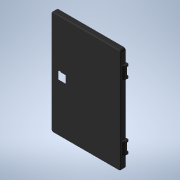
# Autodesk Inventor part: 1301.000_2_(1)
Saved by Autodesk Inventor 2021 (Build 250183000, 183)
## iProperties
Created: 2025-05-02
Part Number: 1301.000_2_(1)
Material: Generic
Catalog Web Link: www.cadenas.de
Description: Deckel KX EB Edelstahl-Deckel KX EB Edelstahl
Vendor: RITTAL
Document SubType Name: Modeling
Designer: psAdmin
Manufacturer: RITTAL
Mass: 142.258 g
Surface Area: 1510.1 cm^2
Volume: 142.258 cm^3
Density: 1 g/cm^3
Appearance: PSOLRGB-175-175-175
Category: PARTsolutions
Company: RITTAL
Title: 1301.000_2
Author: Cadenas PARTsolutions
Comments: Deckel KX EB Edelstahl
PSOL_IDENT_0: {$CADENAS_DATA/23d-libs/rittal/schaltschranksys/edelstahl/kleingehause/parts_eb_edel_2_0/deckel_kx_e
PSOL_IDENT_1: b_edel_new.prj},193 {VTYP=3D},{NB=1301.000_2_(1)},{LINA=1301.000_2},{NN=Deckel KX EB Edelstahl},{DAT
PSOL_IDENT_2: E=28.04.2025 21:10:47},{GEOMDATE=11.04.2025 11:21:28},{VERSION=},{LINEID=690},{WBVAR=DETAIL},{WBNUME
PSOL_IDENT_3: RIC=DETAIL}  {NB=1301.000_2_(1)},{LINA=1301.000_2},{KT=DUMMY},{BEST=1301.000},{DETAIL=1},{B=200},{H=
PSOL_IDENT_4: 300},{W=198.000},{H1=298.000},{A1=167.450},{GEW=3,889},{S1=1.250},{CNSETIM80=EC000261},{CNSETIM90=EC
PSOL_IDENT_5: 000261},{CNSECLASS60=27-18-01-01},{CNSECLASS80=27-18-01-01},{UNSPSC=31-26-15-02}
NB: 1301.000_2_(1)
NN: Deckel KX EB Edelstahl
NT: Deckel KX EB Edelstahl
NBSYN: $BEST._2_($DETAIL.)
LINA: 1301.000_2
CATALOG: Rittal
BEST: 1301.000
DETAIL: hoch
B: 200
H: 300
W: 198
H1: 298
A1: 167.45
GEW: 3,889
S1: 1.25
CNSETIM80: EC000261
CNSETIM90: EC000261
CNSECLASS60: 27-18-01-01
CNSECLASS80: 27-18-01-01
UNSPSC: 31-26-15-02
SUPPLIER: RITTAL
ARTICLENO: 1301.000_2_(1)
BOMINFO: 1301.000_2
CREATOR: CADENAS GmbH
Autodesk Inventor part; units mm, degrees
ref_plane "YZ Plane" through (0, 0, 0) normal (1, 0, 0) x (0, 1, 0)
ref_plane "XZ Plane" through (0, 0, 0) normal (0, 1, 0) x (-1, 0, 0)
ref_plane "XY Plane" through (0, 0, 0) normal (0, 0, 1) x (1, 0, 0)
sketch "Skizze_2" plane through (0, 0, 0) normal (1, 0, 0) x (0, 0, -1)
  line L0 (0, -149) -> (15, -149)
  line L1 (15, -149) -> (15, -147.75)
  line L2 (15, -147.75) -> (1.25, -147.75)
  line L3 (1.25, -147.75) -> (1.25, 147.75)
  line L4 (1.25, 147.75) -> (15, 147.75)
  line L5 (15, 147.75) -> (15, 149)
  line L6 (15, 149) -> (0, 149)
  line L7 (0, 149) -> (0, -149)
  constraints: 16 end point
extrude "Extrusion1" add sketch "Skizze_2" along normal mid plane 186
sketch "Skizze_4" plane through (0, 0, 0) normal (0, 1, 0) x (1, 0, 0)
  line L0 (-99, 15) -> (-99, 0)
  line L1 (-99, 0) -> (99, 0)
  line L2 (99, 0) -> (99, 15)
  line L3 (99, 15) -> (97.75, 15)
  line L4 (97.75, 15) -> (97.75, 1.25)
  line L5 (97.75, 1.25) -> (-97.75, 1.25)
  line L6 (-97.75, 1.25) -> (-97.75, 15)
  line L7 (-97.75, 15) -> (-99, 15)
  constraints: 16 end point
extrude "Extrusion2" add sketch "Skizze_4" along normal mid plane 286
sketch "Skizze_5" plane through (0, 143, 0) normal (0, 1, 0) x (1, 0, 0)
  line L0 (93, 0) -> (93, 1.25)
  line L1 (93, 1.25) -> (97.75, 1.25)
  line L2 (97.75, 1.25) -> (97.75, 15)
  line L3 (97.75, 15) -> (99, 15)
  line L4 (99, 15) -> (99, 2.5)
  arc A0 (96.5, 0) -> (99, 2.5) centre (96.5, 2.5) ccw
  line L5 (96.5, 0) -> (93, 0)
  line L6 (93, 0) -> (93, 1.25)
  constraints: 14 end point, 2 point on circle, 1 centre point
revolve "Revolution1" add sketch "Skizze_5" angle 90 about axis through (93, 143, 0) along (0, 0, 1)
sketch "Skizze_6" plane through (0, 143, 0) normal (0, 1, 0) x (1, 0, 0)
  line L0 (-93, 1.25) -> (-93, 0)
  line L1 (-93, 0) -> (-96.5, 0)
  arc A0 (-99, 2.5) -> (-96.5, 0) centre (-96.5, 2.5) ccw
  line L2 (-99, 2.5) -> (-99, 15)
  line L3 (-99, 15) -> (-97.75, 15)
  line L4 (-97.75, 15) -> (-97.75, 1.25)
  line L5 (-97.75, 1.25) -> (-93, 1.25)
  line L6 (-93, 1.25) -> (-93, 0)
  constraints: 14 end point, 2 point on circle, 1 centre point
revolve "Revolution2" add sketch "Skizze_6" angle 90 about axis through (-93, 143, -1.25) along (0, 0, -1)
sketch "Skizze_7" plane through (0, -143, 0) normal (0, 1, 0) x (1, 0, 0)
  line L0 (93, 0) -> (93, 1.25)
  line L1 (93, 1.25) -> (97.75, 1.25)
  line L2 (97.75, 1.25) -> (97.75, 15)
  line L3 (97.75, 15) -> (99, 15)
  line L4 (99, 15) -> (99, 2.5)
  arc A0 (96.5, 0) -> (99, 2.5) centre (96.5, 2.5) ccw
  line L5 (96.5, 0) -> (93, 0)
  line L6 (93, 0) -> (93, 1.25)
  constraints: 14 end point, 2 point on circle, 1 centre point
revolve "Revolution3" add sketch "Skizze_7" angle 90 about axis through (93, -143, 0) along (0, 0, -1)
sketch "Skizze_8" plane through (0, -143, 0) normal (0, 1, 0) x (1, 0, 0)
  line L0 (-93, 1.25) -> (-93, 0)
  line L1 (-93, 0) -> (-96.5, 0)
  arc A0 (-99, 2.5) -> (-96.5, 0) centre (-96.5, 2.5) ccw
  line L2 (-99, 2.5) -> (-99, 15)
  line L3 (-99, 15) -> (-97.75, 15)
  line L4 (-97.75, 15) -> (-97.75, 1.25)
  line L5 (-97.75, 1.25) -> (-93, 1.25)
  line L6 (-93, 1.25) -> (-93, 0)
  constraints: 14 end point, 2 point on circle, 1 centre point
revolve "Revolution4" add sketch "Skizze_8" angle 90 about axis through (-93, -143, -1.25) along (0, 0, 1)
sketch "Skizze_29" plane through (0, 0, 0) normal (1, 0, 0) x (0, 0, -1)
  line L0 (0, 147.75) -> (0, -147.75)
  line L1 (0, -147.75) -> (1.25, -147.75)
  arc A0 (1.25, -147.75) -> (1.25, -136.75) centre (1.7292, -142.25) ccw
  line L2 (1.25, -136.75) -> (1.25, 136.75)
  arc A1 (1.25, 136.75) -> (1.25, 147.75) centre (1.7292, 142.25) ccw
  line L3 (1.25, 147.75) -> (0, 147.75)
  constraints: 8 end point, 4 point on circle, 2 centre point
extrude "Extrusion3" add sketch "Skizze_29" along normal mid plane 176.5
sketch "Skizze_30" plane through (88.25, 0, 0) normal (1, 0, 0) x (0, 0, -1)
  line L0 (5.5344, 138.25) -> (1.25, 138.25)
  line L1 (1.25, 138.25) -> (1.25, 147.7708)
  line L2 (1.25, 147.7708) -> (1.7292, 147.7708)
  arc A0 (5.5344, 138.25) -> (1.7292, 147.7708) centre (1.7292, 142.25) ccw
  line L3 (5.5344, 138.25) -> (1.25, 138.25)
  constraints: 8 end point, 2 point on circle, 1 centre point
revolve "Revolution5" add sketch "Skizze_30" angle 90 about axis through (88.25, 138.25, -5.5344) along (0, 0, -1)
sketch "Skizze_31" plane through (88.25, 0, 0) normal (1, 0, 0) x (0, 0, -1)
  line L0 (1.25, -138.25) -> (5.5344, -138.25)
  arc A0 (1.7292, -147.7708) -> (5.5344, -138.25) centre (1.7292, -142.25) ccw
  line L1 (1.7292, -147.7708) -> (1.25, -147.7708)
  line L2 (1.25, -147.7708) -> (1.25, -138.25)
  line L3 (1.25, -138.25) -> (5.5344, -138.25)
  constraints: 8 end point, 2 point on circle, 1 centre point
revolve "Revolution6" add sketch "Skizze_31" angle 90 about axis through (88.25, -138.25, -1.25) along (0, 0, 1)
sketch "Skizze_32" plane through (-88.25, 0, 0) normal (1, 0, 0) x (0, 0, -1)
  line L0 (5.5344, 138.25) -> (1.25, 138.25)
  line L1 (1.25, 138.25) -> (1.25, 147.7708)
  line L2 (1.25, 147.7708) -> (1.7292, 147.7708)
  arc A0 (5.5344, 138.25) -> (1.7292, 147.7708) centre (1.7292, 142.25) ccw
  line L3 (5.5344, 138.25) -> (1.25, 138.25)
  constraints: 8 end point, 2 point on circle, 1 centre point
revolve "Revolution7" add sketch "Skizze_32" angle 90 about axis through (-88.25, 138.25, -5.5344) along (0, 0, 1)
sketch "Skizze_33" plane through (-88.25, 0, 0) normal (1, 0, 0) x (0, 0, -1)
  line L0 (1.25, -138.25) -> (5.5344, -138.25)
  arc A0 (1.7292, -147.7708) -> (5.5344, -138.25) centre (1.7292, -142.25) ccw
  line L1 (1.7292, -147.7708) -> (1.25, -147.7708)
  line L2 (1.25, -147.7708) -> (1.25, -138.25)
  line L3 (1.25, -138.25) -> (5.5344, -138.25)
  constraints: 8 end point, 2 point on circle, 1 centre point
revolve "Revolution8" add sketch "Skizze_33" angle 90 about axis through (-88.25, -138.25, -1.25) along (0, 0, -1)
sketch "Skizze_34" plane through (0, 0, 0) normal (0, 1, 0) x (1, 0, 0)
  arc A0 (-86.75, 1.25) -> (-97.75, 1.25) centre (-92.25, 1.7292) ccw
  line L0 (-97.75, 1.25) -> (-97.75, 0)
  line L1 (-97.75, 0) -> (97.75, 0)
  line L2 (97.75, 0) -> (97.75, 1.25)
  arc A1 (97.75, 1.25) -> (86.75, 1.25) centre (92.25, 1.7292) ccw
  line L3 (86.75, 1.25) -> (-86.75, 1.25)
  constraints: 8 end point, 4 point on circle, 2 centre point
extrude "Extrusion4" add sketch "Skizze_34" along normal mid plane 276.5
sketch "Sketch_5" plane through (0, 0, 0) normal (0, 1, 0) x (1, 0, 0)
  line L0 (-109, -10) -> (109, -10)
  line L1 (109, -10) -> (109, 15)
  line L2 (109, 15) -> (99, 15)
  line L3 (99, 15) -> (99, 2.5)
  arc A0 (96.5, 0) -> (99, 2.5) centre (96.5, 2.5) ccw
  line L4 (96.5, 0) -> (-96.5, 0)
  arc A1 (-99, 2.5) -> (-96.5, 0) centre (-96.5, 2.5) ccw
  line L5 (-99, 2.5) -> (-99, 15)
  line L6 (-99, 15) -> (-109, 15)
  line L7 (-109, 15) -> (-109, -10)
  constraints: 16 end point, 4 point on circle, 2 centre point
extrude "Extrusion5" cut sketch "Sketch_5" along normal mid plane 288
sketch "Sketch_6" plane through (0, 0, 0) normal (1, 0, 0) x (0, 0, -1)
  line L0 (-10, -159) -> (15, -159)
  line L1 (15, -159) -> (15, -149)
  line L2 (15, -149) -> (2.5, -149)
  arc A0 (0, -146.5) -> (2.5, -149) centre (2.5, -146.5) ccw
  line L3 (0, -146.5) -> (0, 146.5)
  arc A1 (2.5, 149) -> (0, 146.5) centre (2.5, 146.5) ccw
  line L4 (2.5, 149) -> (15, 149)
  line L5 (15, 149) -> (15, 159)
  line L6 (15, 159) -> (-10, 159)
  line L7 (-10, 159) -> (-10, -159)
  constraints: 16 end point, 4 point on circle, 2 centre point
extrude "Extrusion6" cut sketch "Sketch_6" along normal mid plane 188
sketch "Sketch_3" plane through (0, 0, -1.25) normal (0, 0, 1) x (1, 0, 0)
  arc A0 (-79.6, -10.65) -> (-79.1, -11.15) centre (-79.1, -10.65) ccw
  line L0 (-79.1, -11.15) -> (-57.8, -11.15)
  arc A1 (-57.8, -11.15) -> (-57.3, -10.65) centre (-57.8, -10.65) ccw
  line L1 (-57.3, -10.65) -> (-57.3, 10.65)
  arc A2 (-57.3, 10.65) -> (-57.8, 11.15) centre (-57.8, 10.65) ccw
  line L2 (-57.8, 11.15) -> (-71.1, 11.15)
  arc A3 (-71.6, 11.65) -> (-71.1, 11.15) centre (-71.1, 11.65) ccw
  line L3 (-71.6, 11.65) -> (-71.6, 12.15)
  arc A4 (-71.6, 12.15) -> (-72.1, 12.65) centre (-72.1, 12.15) ccw
  line L4 (-72.1, 12.65) -> (-77.1, 12.65)
  arc A5 (-77.1, 12.65) -> (-77.6, 12.15) centre (-77.1, 12.15) ccw
  line L5 (-77.6, 12.15) -> (-77.6, 11.65)
  arc A6 (-78.1, 11.15) -> (-77.6, 11.65) centre (-78.1, 11.65) ccw
  line L6 (-78.1, 11.15) -> (-79.1, 11.15)
  arc A7 (-79.1, 11.15) -> (-79.6, 10.65) centre (-79.1, 10.65) ccw
  line L7 (-79.6, 10.65) -> (-79.6, -10.65)
  constraints: 16 end point, 16 point on circle, 8 centre point
extrude "Extrusion7" cut sketch "Sketch_3" along normal blind 1.25
sketch "Sketch_1" plane through (0, 0, 0) normal (1, 0, 0) x (0, 0, -1)
  line L0 (13.25, -129) -> (1.25, -129)
  line L1 (1.25, -129) -> (1.25, -125.25)
  line L2 (1.25, -125.25) -> (2.45, -125.25)
  line L3 (2.45, -125.25) -> (2.45, -126)
  arc A0 (2.45, -126) -> (2.95, -126.5) centre (2.95, -126) ccw
  line L4 (2.95, -126.5) -> (3.95, -126.5)
  arc A1 (3.95, -126.5) -> (4.45, -126) centre (3.95, -126) ccw
  line L5 (4.45, -126) -> (12.6365, -126)
  line L6 (12.6365, -126) -> (13.25, -126.6135)
  line L7 (13.25, -126.6135) -> (13.25, -129)
  line L8 (13.25, -129) -> (1.25, -129)
  constraints: 18 end point, 4 point on circle, 2 centre point
revolve "Revolution9" add sketch "Sketch_1" angle 360 about axis through (0, -129, -13.25) along (0, 0, -1)
thread "Thread1" size "M6x1" class "6g" standard "ISO Metric profile" length 7.1865
sketch "Sketch_4" plane through (0, 93.5, 0) normal (0, 1, 0) x (1, 0, 0)
  arc A0 (95, 10.5) -> (95.5, 10) centre (95.5, 10.5) ccw
  line L0 (95.5, 10) -> (96.8, 10)
  arc A1 (96.8, 10) -> (97.3, 10.5) centre (96.8, 10.5) ccw
  line L1 (97.3, 10.5) -> (97.3, 15)
  line L2 (97.3, 15) -> (99, 15)
  line L3 (99, 15) -> (99, 3)
  line L4 (99, 3) -> (99.756, 3)
  arc A2 (99.756, 3) -> (100.1501, 3.1923) centre (99.756, 3.5) ccw
  line L5 (100.1501, 3.1923) -> (104, 8.1235)
  line L6 (104, 8.1235) -> (104.4949, 15.84)
  arc A3 (104.4949, 15.84) -> (102, 18.5) centre (102, 16) ccw
  line L7 (102, 18.5) -> (97.2071, 18.5)
  arc A4 (97.2071, 18.5) -> (96.8536, 18.3536) centre (97.2071, 18) ccw
  line L8 (96.8536, 18.3536) -> (95.1464, 16.6464)
  arc A5 (95.1464, 16.6464) -> (95, 16.2929) centre (95.5, 16.2929) ccw
  line L9 (95, 16.2929) -> (95, 10.5)
  circle A6 centre (102, 16) radius 1.25
  constraints: 20 end point, 12 point on circle, 7 centre point
extrude "Extrusion8" add sketch "Sketch_4" along normal mid plane 35
sketch "Sketch_10" plane through (0, -93.5, 0) normal (0, 1, 0) x (1, 0, 0)
  arc A0 (95, 10.5) -> (95.5, 10) centre (95.5, 10.5) ccw
  line L0 (95.5, 10) -> (96.8, 10)
  arc A1 (96.8, 10) -> (97.3, 10.5) centre (96.8, 10.5) ccw
  line L1 (97.3, 10.5) -> (97.3, 15)
  line L2 (97.3, 15) -> (99, 15)
  line L3 (99, 15) -> (99, 3)
  line L4 (99, 3) -> (99.756, 3)
  arc A2 (99.756, 3) -> (100.1501, 3.1923) centre (99.756, 3.5) ccw
  line L5 (100.1501, 3.1923) -> (104, 8.1235)
  line L6 (104, 8.1235) -> (104.4949, 15.84)
  arc A3 (104.4949, 15.84) -> (102, 18.5) centre (102, 16) ccw
  line L7 (102, 18.5) -> (97.2071, 18.5)
  arc A4 (97.2071, 18.5) -> (96.8536, 18.3536) centre (97.2071, 18) ccw
  line L8 (96.8536, 18.3536) -> (95.1464, 16.6464)
  arc A5 (95.1464, 16.6464) -> (95, 16.2929) centre (95.5, 16.2929) ccw
  line L9 (95, 16.2929) -> (95, 10.5)
  circle A6 centre (102, 16) radius 1.25
  constraints: 20 end point, 12 point on circle, 7 centre point
extrude "Extrusion9" add sketch "Sketch_10" along normal mid plane 35
sketch "Sketch_9" plane through (0, -93.5, 0) normal (0, 1, 0) x (1, 0, 0)
  arc A0 (95, 10.5) -> (95.5, 10) centre (95.5, 10.5) ccw
  line L0 (95.5, 10) -> (96.8, 10)
  arc A1 (96.8, 10) -> (97.3, 10.5) centre (96.8, 10.5) ccw
  line L1 (97.3, 10.5) -> (97.3, 15)
  line L2 (97.3, 15) -> (99, 15)
  line L3 (99, 15) -> (99, 13.3)
  line L4 (99, 13.3) -> (104.332, 13.3)
  line L5 (104.332, 13.3) -> (104.4949, 15.84)
  arc A2 (104.4949, 15.84) -> (102, 18.5) centre (102, 16) ccw
  line L6 (102, 18.5) -> (97.2071, 18.5)
  arc A3 (97.2071, 18.5) -> (96.8536, 18.3536) centre (97.2071, 18) ccw
  line L7 (96.8536, 18.3536) -> (95.1464, 16.6464)
  arc A4 (95.1464, 16.6464) -> (95, 16.2929) centre (95.5, 16.2929) ccw
  line L8 (95, 16.2929) -> (95, 10.5)
  constraints: 18 end point, 10 point on circle, 5 centre point
extrude "Extrusion10" cut sketch "Sketch_9" along normal mid plane 25
sketch "Sketch_11" plane through (0, 93.5, 0) normal (0, 1, 0) x (1, 0, 0)
  arc A0 (95, 10.5) -> (95.5, 10) centre (95.5, 10.5) ccw
  line L0 (95.5, 10) -> (96.8, 10)
  arc A1 (96.8, 10) -> (97.3, 10.5) centre (96.8, 10.5) ccw
  line L1 (97.3, 10.5) -> (97.3, 15)
  line L2 (97.3, 15) -> (99, 15)
  line L3 (99, 15) -> (99, 13.3)
  line L4 (99, 13.3) -> (104.332, 13.3)
  line L5 (104.332, 13.3) -> (104.4949, 15.84)
  arc A2 (104.4949, 15.84) -> (102, 18.5) centre (102, 16) ccw
  line L6 (102, 18.5) -> (97.2071, 18.5)
  arc A3 (97.2071, 18.5) -> (96.8536, 18.3536) centre (97.2071, 18) ccw
  line L7 (96.8536, 18.3536) -> (95.1464, 16.6464)
  arc A4 (95.1464, 16.6464) -> (95, 16.2929) centre (95.5, 16.2929) ccw
  line L8 (95, 16.2929) -> (95, 10.5)
  constraints: 18 end point, 10 point on circle, 5 centre point
extrude "Extrusion11" cut sketch "Sketch_11" along normal mid plane 25
ref_plane "DECKEL_XY" through (0, 0, 0) normal (0, 0, -1) x (1, 0, 0)
ref_plane "DECKEL_YZ" through (0, 0, 0) normal (1, 0, 0) x (0, -1, 0)
ref_plane "DECKEL_ZX" through (0, 0, 0) normal (0, -1, 0) x (0, 0, -1)
ref_plane "VB_XY" through (-68.45, 0, 0) normal (0, 0, -1) x (1, 0, 0)
ref_plane "VB_YZ" through (-68.45, 0, 0) normal (1, 0, 0) x (0, -1, 0)
ref_plane "VB_ZX" through (-68.45, 0, 0) normal (0, -1, 0) x (0, 0, -1)
ref_plane "to_HINGE_XY" through (102, 93.5, -16) normal (0, 1, 0) x (1, 0, 0)
ref_plane "to_HINGE_YZ" through (102, 93.5, -16) normal (1, 0, 0) x (0, 0, -1)
ref_plane "to_HINGE_ZX" through (102, 93.5, -16) normal (0, 0, -1) x (0, 1, 0)
ref_plane "to_HINGE_1_XY" through (102, -93.5, -16) normal (0, 1, 0) x (1, 0, 0)
ref_plane "to_HINGE_1_YZ" through (102, -93.5, -16) normal (1, 0, 0) x (0, 0, -1)
ref_plane "to_HINGE_1_ZX" through (102, -93.5, -16) normal (0, 0, -1) x (0, 1, 0)
body "Solid1"
